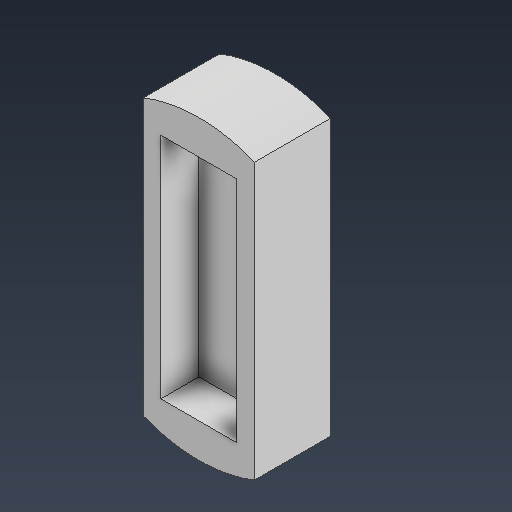
# Autodesk Inventor part: Sorting Gate Edited
Saved by Autodesk Inventor 2025.3 (Build 293356000, 356)
## iProperties
Created: 2026-04-15
Part Number: Sorting Gate Edited
Material: Generic
Document SubType Name: Modeling
Designer: manon
Density: 1 g/cm^3
Appearance: Default
Author: manon
Autodesk Inventor part; units mm, degrees
ref_plane "YZ Plane" through (0, 0, 0) normal (1, 0, 0) x (0, 1, 0)
ref_plane "XZ Plane" through (0, 0, 0) normal (0, 1, 0) x (-1, 0, 0)
ref_plane "XY Plane" through (0, 0, 0) normal (0, 0, 1) x (1, 0, 0)
sketch "Sketch1" plane through (0, 0, 0) normal (0, 0, 1) x (1, 0, 0)
  circle A0 centre (0, 0) radius 58.5
  line L0 (0, 0) -> (0, 58.5) construction
  line L1 (0, 0) -> (-58.5, 0) construction
  line L2 (-21.9335, 54.2326) -> (-21.9335, -54.2326)
  line L3 (21.9335, 54.2326) -> (21.9335, -54.2326)
  point P0 (-54.2326, 21.9335)
  point P1 (54.2326, 21.9335)
  dimension "d0" = 117
  dimension "d53" = 21.9335
  constraints: 8 end point, 2 vertical, 1 coincident, 1 horizontal, 10 other
  measures "d53" distance between parallel lines of L0 L2
extrude "Extrusion1" add sketch "Sketch1" along normal blind 30 contours L3 A0 L2
sketch "Sketch2" plane through (0, 0, 0) normal (0, 0, -1) x (-1, 0, 0)
  circle A0 centre (0, 0) radius 6.5
  dimension "d4" = 13
  constraints: 1 centre point, 1 coincident
  measures "d4" diameter of A0
extrude "Extrusion2" add sketch "Sketch2" along normal blind 15
sketch "Sketch6" plane through (0, 0, -15) normal (0, 0, -1) x (-1, 0, 0)
  circle A0 centre (0, 0) radius 1.15
  circle A1 centre (0, 0) radius 1.15
  line L0 (18.75, 0) -> (16.35, 0) construction
  line L1 (16.35, 0) -> (0, 0) construction
  line L2 (0, 0) -> (0, 3.75) construction
  circle A2 centre (0, 0) radius 3.9
  circle A3 centre (16.35, 0) radius 2.55
  line L3 (16.35, 2.55) -> (0.3241, 3.8865)
  line L4 (16.35, -2.55) -> (0.3241, -3.8865)
  point P0 (0, 3.75)
  dimension "d21" = 2.4
  dimension "d24" = 2.3
  dimension "d27" = 7.8
  dimension "d28" = 5.1
  dimension "d29" = 16.0259
  dimension "d30" = 16.0259
  constraints: 10 end point, 4 centre point, 4 point on circle, 2 coincident, 2 tangent, 1 collinear, 1 concentric, 1 horizontal
  measures "d21" distance of L0.start L0.end
  measures "d24" diameter of A0
  measures "d27" diameter of A2
  measures "d28" diameter of A3
  measures "d29" horizontal distance of L3.start L3.end
  measures "d30" horizontal distance of L4.start L4.end
extrude "Extrusion5" [suppressed]
sketch "Sketch7" plane through (0, 0, -12.2) normal (0, 0, -1) x (-1, 0, 0)
  circle A0 centre (0, 0) radius 1.15
  dimension "d33" = 2.3
  constraints: 1 centre point, 1 coincident
  measures "d33" diameter of A0
extrude "Extrusion6" [suppressed]
sketch "Sketch8" plane through (0, 0, 30) normal (0, 0, 1) x (1, 0, 0)
  line L0 (0, 0) -> (21.9335, 0) construction
  line L1 (0, 0) -> (15, 0)
  line L2 (15, 0) -> (15, 45)
  line L3 (15, 45) -> (-15, 45)
  line L4 (-15, 45) -> (-15, 0)
  line L5 (-15, 0) -> (0, 0)
  line L6 (-15, 0) -> (-15, -45)
  line L7 (-15, -45) -> (15, -45)
  line L8 (15, -45) -> (15, 0)
  dimension "d43" = 15
  dimension "d44" = 45
  dimension "d45" = 30
  dimension "d46" = 45
  dimension "d47" = 30
  constraints: 18 end point, 3 perpendicular, 3 point on line
  measures "d43" distance of L1.start L1.end
  measures "d44" distance of L1.end L2.end
  measures "d45" distance of L2.end L3.end
  measures "d46" distance of L4.end L6.end
  measures "d47" distance of L6.end L7.end
extrude "Extrusion7" cut sketch "Sketch8" against normal blind 15
sketch "Sketch9" plane through (0, 0, -15) normal (0, 0, -1) x (-1, 0, 0)
  circle A0 centre (0, 0) radius 3.5
  arc A1 (1.9, 14.1) -> (-1.8987, 14.0987) centre (0.0007, 14.05) ccw
  line L0 (0.0007, 15.95) -> (0.0007, 14.05)
  line L1 (0.0007, 14.05) -> (0, 0)
  circle A2 centre (0.0007, 14.05) radius 1.9
  line L2 (-1.8987, 14.0987) -> (-2.75, 2.1651)
  line L3 (-2.75, 2.1651) -> (-1.8987, 14.0987)
  line L4 (2.75, 2.1651) -> (1.9, 14.1)
  line L5 (2.75, 2.1651) -> (1.9, 14.1)
  constraints: 12 end point, 3 centre point, 3 coincident, 3 point on circle, 2 collinear, 1 concentric, 1 vertical
extrude "Extrusion8" cut sketch "Sketch9" against normal blind 3.8
sketch "Sketch10" plane through (0, 0, -11.2) normal (0, 0, -1) x (-1, 0, 0)
  circle A0 centre (0, 0) radius 1.15
  dimension "d50" = 2.3
  constraints: 1 centre point, 1 coincident
  measures "d50" diameter of A0
extrude "Extrusion9" add sketch "Sketch10" along normal blind 3
body "Solid1"
